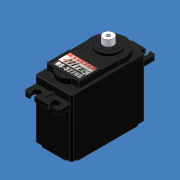
# Autodesk Inventor part: Hitec Servo
Saved by Autodesk Inventor 2012 (Build 160160000, 160)
## iProperties
Shininess: 64.0
Length Units: 11269
Angle Units: 11279
Time Units: 11290
Mass Units: 11283
Length Display Precision: 3
Angle Display Precision: 2
Compacted: True
Part Number: Hitec Servo
Document SubType Name: Modeling
Created: 2006-01-15
Designer: Ed Sparks
Material: ABS Plastic
Density: 1 g/cm^3
Density: 0.0
Volumn: 0.0
Area: 0.0
PropertySet Name: Model Information
Control State: 0
Master: False
Checked Out: False
Author: Ed Sparks
Autodesk Inventor part; units mm, degrees
ref_plane "YZ Plane" through (0, 0, 0) normal (1, 0, 0) x (0, 1, 0)
ref_plane "XZ Plane" through (0, 0, 0) normal (0, 1, 0) x (-1, 0, 0)
sketch "Sketch1" plane through (0, 0, 0) normal (0, 0, 1) x (1, 0, 0)
  line L0 (-20, 10) -> (20, 10)
  line L1 (20, 10) -> (20, -10)
  line L2 (20, -10) -> (-20, -10)
  line L3 (-20, -10) -> (-20, 10)
  line L4 (0, 0) -> (0, 10) construction
  line L5 (0, 0) -> (0, -10) construction
  line L6 (0, 0) -> (20, 0) construction
  line L7 (0, 0) -> (-20, 0) construction
  dimension "d0" = 40
  dimension "d1" = 20
  constraints: 16 end point, 4 midpoint, 4 perpendicular, 3 parallel, 2 collinear, 1 horizontal, 1 other
  measures "d0" distance of L0.start L0.end
  measures "d1" distance of L0.end L1.end
extrude "Extrusion1" add sketch "Sketch1" along normal blind 33
sketch "Sketch2" plane through (0, 0, 33) normal (0, 0, 1) x (1, 0, 0)
  line L0 (20, 10) -> (20, -10) projected
  line L1 (-20, -10) -> (-20, 10) projected
  line L2 (-7.2207, 8.875) -> (14.8541, 8.875)
  line L3 (14.8541, -8.875) -> (-7.2207, -8.875)
  line L4 (0, 0) -> (0, 8.875) construction
  line L5 (0, 0) -> (0, -8.875) construction
  arc A0 (-7.2207, 8.875) -> (-7.2207, -8.875) centre (-10, 0) ccw
  arc A1 (14.8541, -4.875) -> (14.8541, 4.875) centre (11, 0) ccw
  line L6 (14.8541, 8.875) -> (14.8541, 4.875)
  line L7 (14.8541, -4.875) -> (14.8541, -8.875)
  dimension "d4" = 17.75
  dimension "d6" = 18.6
  dimension "d7" = 10
  dimension "d11" = 4
  dimension "d12" = 9
  constraints: 12 end point, 4 point on circle, 3 perpendicular, 2 centre point, 2 collinear, 2 horizontal alignment, 2 point on line, 1 horizontal, 1 parallel, 1 other
  measures "d4" distance of L2.end L3.start
  measures "d6" diameter of A0
  measures "d7" distance from line of A0.centre L1
  measures "d11" distance of L2.end L6.end
  measures "d12" distance from line of L0 A1.centre
extrude "Extrusion2" add sketch "Sketch2" along normal blind 3
sketch "Sketch3" plane through (0, 0, 36) normal (0, 0, 1) x (1, 0, 0)
  arc A0 (-7.2207, 8.875) -> (-7.2207, -8.875) centre (-10, 0) ccw projected
  circle A1 centre (-10, 0) radius 6.45
  dimension "d13" = 12.9
  constraints: 1 centre point, 1 coincident, 1 concentric
  measures "d13" diameter of A1
extrude "Extrusion3" add sketch "Sketch3" along normal blind 1.5
sketch "Sketch4" plane through (-10, 0, 37.5) normal (0, 0, 1) x (1, 0, 0)
  circle A0 centre (0, 0) radius 6.45 projected
  circle A1 centre (0, 0) radius 4.975
  dimension "d16" = 9.95
  constraints: 1 centre point, 1 coincident, 1 concentric
  measures "d16" diameter of A1
extrude "Extrusion4" add sketch "Sketch4" along normal blind 0.5 contours A1
ref_plane "Work Plane1" through (0, 0, 26.5) normal (0, 0, -1) x (-1, 0, 0)
sketch "Sketch5" plane through (0, 0, 26.5) normal (0, 0, -1) x (-1, 0, 0)
  line L0 (-20, 10) -> (-20, -10) projected
  line L1 (-20, -10) -> (20, -10) projected
  line L2 (-20, 10) -> (-20, -10) projected
  line L3 (-20, 10) -> (-20, -10) projected
  line L4 (20, 10) -> (-20, 10) projected
  line L5 (-20, -9.45) -> (-26.4, -9.45)
  line L6 (-26.4, -9.45) -> (-26.4, 9.45)
  line L7 (-26.4, 9.45) -> (-20, 9.45)
  line L8 (-20, 9.45) -> (-20, -9.45)
  line L9 (-20, -10) -> (-20, -9.45) construction
  line L10 (-20, 9.45) -> (-20, 10) construction
  dimension "d20" = 18.9
  dimension "d21" = 6.4
  constraints: 12 end point, 3 collinear, 2 parallel, 2 perpendicular, 1 horizontal
  measures "d20" distance of L5.end L6.end
  measures "d21" distance of L6.end L7.end
extrude "Extrusion5" add sketch "Sketch5" against normal blind 2.5
sketch "Sketch6" plane through (0, 0, 29) normal (0, 0, 1) x (1, 0, 0)
  line L0 (20, -9.45) -> (20, 9.45) projected
  line L1 (26.4, 9.45) -> (26.4, -9.45) projected
  line L2 (20, 9.45) -> (26.4, 9.45) projected
  circle A0 centre (-10, 0) radius 4.975 projected
  arc A1 (25.6748, 6.4) -> (25.6748, 3.8) centre (23.9, 5.1) ccw
  line L3 (25.6748, 6.4) -> (26.4, 6.4)
  line L4 (25.6748, 3.8) -> (26.4, 3.8)
  dimension "d26" = 3.9
  dimension "d27" = 5.1
  dimension "d28" = 4.4
  dimension "d29" = 2.6
  constraints: 4 end point, 3 parallel, 2 point on circle, 2 point on line, 1 centre point
  measures "d26" distance from line of A1.centre L0
  measures "d27" vertical distance of A1.centre A0.centre
  measures "d28" diameter of A1
  measures "d29" distance between parallel lines of L4 L3
extrude "Extrusion6" cut sketch "Sketch6" against normal through all contours L1 L4 A1 L3
mirror "Mirror2" about plane through (0, 0, 0) normal (0, 1, 0) of "Extrusion6"
sketch "Sketch7" plane through (0, 0, 29) normal (0, 0, 1) x (1, 0, 0)
  line L0 (20, -9.45) -> (20, 9.45) projected
  line L1 (20, 10) -> (20, -10) projected
  line L2 (20, 0.58) -> (23.42, 0.58)
  line L3 (24, 0) -> (24, 0)
  line L4 (23.42, -0.58) -> (20, -0.58)
  line L5 (20, -0.58) -> (20, 0.58)
  circle A0 centre (-10, 0) radius 4.975 projected
  line L6 (-10, 0) -> (32.8804, 0) construction
  line L7 (20, 0) -> (20, 0.58) construction
  line L8 (20, 0) -> (20, -0.58) construction
  arc A1 (24, 0) -> (23.42, 0.58) centre (23.42, 0) ccw
  arc A2 (23.42, -0.58) -> (24, 0) centre (23.42, 0) ccw
  point P0 (24, -0.58)
  point P1 (24, 0.58)
  dimension "d33" = 1.16
  dimension "d34" = 4
  dimension "d35" = 0.58
  constraints: 14 end point, 5 point on line, 4 collinear, 4 point on circle, 4 tangent, 2 centre point, 2 parallel, 2 perpendicular, 1 concentric, 1 horizontal, 1 midpoint
  measures "d33" distance of point (24, 0.58) point (24, -0.58)
  measures "d34" distance of point (24, -0.58) L4.end
  measures "d35" radius of A1
extrude "Extrusion7" add sketch "Sketch7" along normal blind 0.9 contours L0 L2 A1 A2 L4
mirror "Mirror3" about plane through (0, 0, 0) normal (1, 0, 0) of "Extrusion6", "Extrusion5", "Mirror2", "Extrusion7"
fillet "Fillet2" radius 1 4 edges at (-26.4, -9.45, 27.75) (-26.4, 9.45, 27.75) (26.4, 9.45, 27.75) (26.4, -9.45, 27.75)
sketch "Sketch8" plane through (0, 0, 0) normal (0, 0, -1) x (-1, 0, 0)
  line L0 (-20, 10) -> (-16, 10)
  line L1 (-16, 10) -> (-16, 6)
  line L2 (-16, 6) -> (-20, 6)
  line L3 (-20, 6) -> (-20, 10)
  dimension "d39" = 4
  constraints: 8 end point, 2 parallel, 2 perpendicular, 1 horizontal
  measures "d39" distance of L0.end L1.end
extrude "Extrusion8" cut sketch "Sketch8" against normal blind 1.5
sketch "Sketch12" plane through (0, 0, 1.5) normal (0, 0, -1) x (-1, 0, 0)
  line L0 (-20, 6) -> (-20, 10) projected
  line L1 (20, 10) -> (-16, 10) projected
  point P0 (-18, 8)
  dimension "d64" = 2
  dimension "d65" = 2
  measures "d64" distance from line of point (-18, 8) L1
  measures "d65" distance from line of L0 point (-18, 8)
hole "Hole1" at (18, 8, 1.5) direction (0, 0, 1) diameter 1.8 depth 8 tip angle 118
mirror "Mirror4" about plane through (0, 0, 0) normal (1, 0, 0) of "Extrusion8", "Hole1"
mirror "Mirror5" about plane through (0, 0, 0) normal (0, 1, 0) of "Extrusion8", "Mirror4", "Hole1"
fillet "Fillet4" radius 2 4 edges at (-16, 6, 0.75) (-16, -6, 0.75) (16, 6, 0.75) (16, -6, 0.75)
chamfer "Chamfer1" distance 0.25 angle 45 4 edges at (0, -10, 33) (20, 0, 33) (0, 10, 33) (-20, 0, 33)
fillet "Fillet5" radius 1 4 edges at (20, -10, 17.125) (-20, -10, 17.125) (-20, 10, 17.125) (20, 10, 17.125)
chamfer "Chamfer2" distance 0.75 angle 45 4 edges at (0, -10, 0) (-20, 0, 0) (0, 10, 0) (20, 0, 0)
sketch "Sketch9" plane through (-10, 0, 38) normal (0, 0, 1) x (1, 0, 0)
  circle A0 centre (0, 0) radius 4.975 projected
  circle A1 centre (0, 0) radius 2.85
  circle A2 centre (0, 0) radius 1
  dimension "d49" = 5.7
  dimension "d52" = 2
  constraints: 2 centre point, 2 coincident, 2 concentric
  measures "d49" diameter of A1
  measures "d52" diameter of A2
extrude "Extrusion9" add sketch "Sketch9" along normal blind 3.4 contours A1
fillet "Fillet6" radius 0.5 2 edges at (14.8541, -8.875, 34.5) (14.8541, 8.875, 34.5)
sketch "Sketch10" plane through (0, 0, 36) normal (0, 0, 1) x (1, 0, 0)
  arc A0 (14.8541, 8.375) -> (14.3541, 8.875) centre (14.3541, 8.375) ccw projected
  line L0 (-7.2207, 8.875) -> (14.3541, 8.875) projected
  line L1 (14.3541, -8.875) -> (-7.2207, -8.875) projected
  arc A1 (14.3541, -8.875) -> (14.8541, -8.375) centre (14.3541, -8.375) ccw projected
  line L2 (14.8541, -4.875) -> (14.8541, -8.375) projected
  arc A2 (14.8541, -4.875) -> (14.8541, 4.875) centre (11, 0) ccw projected
  line L3 (14.8541, 8.375) -> (14.8541, 4.875) projected
  line L4 (14.8541, 4.875) -> (14.8541, -4.875)
  circle A3 centre (-10, 0) radius 4.975 projected
  arc A4 (2.0041, 2) -> (2.0041, -2) centre (2.0041, 0) ccw
  line L5 (2.0041, 8.875) -> (2.0041, 2)
  line L6 (2.0041, -2) -> (2.0041, -8.875)
  dimension "d55" = 4
  constraints: 6 end point, 2 parallel, 2 point on circle, 2 point on line, 1 centre point, 1 collinear, 1 horizontal alignment
  measures "d55" diameter of A4
extrude "Extrusion10" add sketch "Sketch10" along normal blind 0.5 contours L3 L4 L2 A1 L1 L6 A4 L5 L0 A0
fillet "Fillet7" radius 0.5 2 edges at (2.0041, 8.875, 36.25) (2.0041, -8.875, 36.25)
sketch "Sketch11" plane through (0, 0, 36.5) normal (0, 0, 1) x (1, 0, 0)
  line L0 (14.3541, -8.875) -> (2.5041, -8.875) projected
  line L1 (14.8541, 8.375) -> (14.8541, -8.375) projected
  line L2 (2.5041, 8.875) -> (14.3541, 8.875) projected
  line L3 (2.0041, 2) -> (2.0041, 8.375) projected
  line L4 (3.0041, 7.875) -> (13.8541, 7.875)
  line L5 (13.8541, 7.875) -> (13.8541, -7.875)
  line L6 (13.8541, -7.875) -> (3.0041, -7.875)
  line L7 (3.0041, -7.875) -> (3.0041, 7.875)
  line L8 (3.0041, 7.875) -> (2.0041, 7.875) construction
  line L9 (13.8541, -7.875) -> (14.8541, -7.875) construction
  dimension "d59" = 1
  dimension "d60" = 1
  dimension "d61" = 1
  constraints: 12 end point, 3 parallel, 3 perpendicular, 2 point on line, 1 horizontal
  measures "d59" distance between parallel lines of L2 L4
  measures "d60" distance between parallel lines of L1 L5
  measures "d61" distance between parallel lines of L0 L6
extrude "Extrusion11" cut sketch "Sketch11" against normal blind 0.5
decal "Decal1"
sketch "Sketch13" plane through (0, 0, 36) normal (0, 0, 1) x (1, 0, 0)
  line L0 (3.0041, 7.875) -> (3.0041, -7.875) projected
  line L1 (3.0041, -7.875) -> (13.8541, -7.875) projected
  line L2 (13.8541, 7.875) -> (3.0041, 7.875) projected
  line L3 (3.0041, -7.875) -> (3.0041, 7.875) construction
  line L4 (3.0041, 7.875) -> (14.1415, 7.875) construction
  line L5 (14.1415, 7.875) -> (14.1415, -7.875) construction
  line L6 (14.1415, -7.875) -> (3.0041, -7.875) construction
  constraints: 3 collinear, 2 other
body "Solid1"
